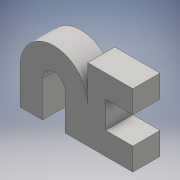
# Autodesk Inventor part: rubber_band_hook
Saved by Autodesk Inventor 2016 (Build 200138000, 138)
## iProperties
Created: 2017-06-18
Part Number: rubber_band_hook
Material: Generic
Document SubType Name: Modeling
Designer: ajar021
Density: 1 g/cm^3
Appearance: Default
Author: ajar021
Autodesk Inventor part; units mm, degrees
ref_plane "YZ Plane" through (0, 0, 0) normal (1, 0, 0) x (0, 1, 0)
ref_plane "XZ Plane" through (0, 0, 0) normal (0, 1, 0) x (-1, 0, 0)
ref_plane "XY Plane" through (0, 0, 0) normal (0, 0, 1) x (1, 0, 0)
sketch "Sketch1" plane through (0, 0, 0) normal (0, 1, 0) x (-1, 0, 0)
  line L0 (0, 0) -> (0, -3)
  line L1 (0, -3) -> (-3, -3)
  line L2 (0, 0) -> (-3, 0)
  line L3 (-3, 0) -> (-3, 2.5)
  line L4 (-3, 2.5) -> (2, 2.5)
  line L5 (2, 2.5) -> (2, 0)
  line L6 (-3, -3) -> (-3, -5.5)
  line L7 (-3, -5.5) -> (4.5, -5.5)
  line L8 (4.5, -5.5) -> (4.5, -1.5)
  arc A0 (7, -1.5) -> (4.5, -1.5) centre (5.75, -1.5) ccw
  line L9 (7, -1.5) -> (7, -5.5)
  line L10 (7, -5.5) -> (9.5, -5.5)
  line L11 (9.5, -5.5) -> (9.5, -1.5)
  line L12 (2, 0) -> (2, -1.5)
  line L13 (4.5, -1.5) -> (2, -1.5) construction
  arc A1 (9.5, -1.5) -> (2, -1.5) centre (5.75, -1.5) ccw
  line L14 (2, -1.5) -> (2, -1.5)
  dimension "d0" = 3
  dimension "d1" = 3
  dimension "d2" = 2.5
  dimension "d3" = 5
  dimension "d4" = 2.5
  dimension "d5" = 7.5
  dimension "d6" = 2.5
  dimension "d7" = 1.25
  dimension "d8" = 2.5
  dimension "d9" = 2.5
  dimension "d10" = 3
  dimension "d13" = 0
  dimension "d14" = 2
  constraints: 30 end point, 7 perpendicular, 5 vertical, 4 point on circle, 3 horizontal, 2 centre point, 1 point on line, 1 tangent
  measures "d0" distance of L0.start L0.end
  measures "d1" distance of L0.end L1.end
  measures "d2" distance of L2.end L3.end
  measures "d3" distance of L3.end L4.end
  measures "d4" distance of L1.end L6.end
  measures "d5" distance of L6.end L7.end
  measures "d6" distance of L8.end L9.start
  measures "d7" radius of A0
  measures "d8" distance of L9.end L10.end
  measures "d9" distance of L8.end L13.end
  measures "d10" distance of L0.start L2.end
  measures "d13" distance of L12.end L13.end
  measures "d14" distance of L5.end L0.start
extrude "Extrusion1" add sketch "Sketch1" along normal blind 3
equation "\"d2\" = d4"
equation "\"d8\" = d4"
equation "\"d10\" = d1"
body "Solid1"
